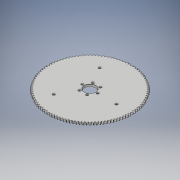
# Autodesk Inventor part: engrenage_rotation
Saved by Autodesk Inventor 2019 (Build 230136000, 136)
## iProperties
Created: 2018-05-17
Part Number: engrenage_rotation
Material: Générique
Document SubType Name: Modeling
Designer: Theo
Density: 1 g/cm^3
Appearance: Par défaut
Author: Theo
Autodesk Inventor part; units mm, degrees
ref_plane "YZ Plane" through (0, 0, 0) normal (1, 0, 0) x (0, 1, 0)
ref_plane "XZ Plane" through (0, 0, 0) normal (0, 1, 0) x (-1, 0, 0)
ref_plane "XY Plane" through (0, 0, 0) normal (0, 0, 1) x (1, 0, 0)
sketch "Esquisse1" plane through (0, 0, 0) normal (1, 0, 0) x (0, 1, 0)
  line L0 (-18.9677, 0) -> (18.9677, 0)
  line L1 (0, 99.5) -> (-0.5, 100)
  line L2 (-0.5, 100) -> (-4.5, 100)
  line L3 (-4.5, 100) -> (-5, 99.5)
  line L4 (-5, 99.5) -> (-5, 13.5)
  line L5 (0, 99.5) -> (0, 14)
  line L6 (-5, 13.5) -> (-0.5, 13.5)
  line L7 (0, 14) -> (-0.5, 13.5)
  point P0 (0, 0)
  point P1 (0, 0)
  dimension "d0" = 0.5
  dimension "d1" = 0.5
  dimension "d2" = 0.5
  dimension "d3" = 0.5
  dimension "d17" = 200
  dimension "d18" = 0.5
  dimension "d19" = 0.5
  dimension "d20" = 27
  dimension "d21" = 5
  constraints: 16 end point, 3 horizontal, 2 vertical, 1 coincident, 1 midpoint, 1 vertical alignment
  measures "d0" horizontal distance of L1.start L1.end
  measures "d1" horizontal distance of L1.start L1.end
  measures "d2" horizontal distance of L2.end L3.end
  measures "d3" horizontal distance of L2.end L3.end
  measures "d17" diameter of L2 L0
  measures "d18" horizontal distance of L5.end L6.end
  measures "d19" horizontal distance of L5.end L6.end
  measures "d20" diameter of L6 L0
  measures "d21" distance between parallel lines of L5 L4
revolve "Révolution1" add sketch "Esquisse1" angle 360 about axis through (0, -18.9677, 0) along (0, 1, 0)
sketch "Esquisse2" plane through (0, 0, 0) normal (0, 1, 0) x (1, 0, 0)
  point P0 (0, 0)
  point P1 (18.25, 0)
  point P2 (9.125, 15.805)
  point P3 (-9.125, 15.805)
  point P4 (-18.25, 0)
  point P5 (-9.125, -15.805)
  point P6 (9.125, -15.805)
  point P7 (63, 0)
  point P8 (-31.5, 54.5596)
  point P9 (-31.5, -54.5596)
  dimension "d23" = 18.25
  dimension "d26" = 360
  dimension "d44" = 63
  dimension "d47" = 360
  constraints: 2 horizontal alignment, 11 other
  measures "d23" distance of point (0, 0) point (18.25, 0)
  measures "d44" distance of point (63, 0) point (0, 0)
hole "Perçage1" at (18.25, 0, 0) at (9.125, 0, -15.805) at (-9.125, 0, -15.805) at (-18.25, 0, 0) at (-9.125, 0, 15.805) at (9.125, 0, 15.805) at (-31.5, 0, 54.5596) at (-31.5, 0, -54.5596) at (63, 0, 0) direction (0, -1, 0) diameter 4.2 end through all counterbore diameter 6 counterbore depth 2
sketch "Esquisse3" plane through (0, 0, 0) normal (0, 1, 0) x (1, 0, 0)
  line L0 (-2.43, -99.7088) -> (-0.433, -96.25)
  arc A0 (0.433, -96.25) -> (-0.433, -96.25) centre (0, -96.5) ccw
  line L1 (0.433, -96.25) -> (2.43, -99.7088)
  arc A1 (2.43, -99.7088) -> (2.8774, -99.9586) centre (2.863, -99.4588) ccw
  arc A2 (-2.8774, -99.9586) -> (-2.43, -99.7088) centre (-2.863, -99.4588) ccw
  circle A3 centre (0, 0) radius 100 projected
  circle A4 centre (0, 0) radius 99.5 projected
  circle A5 centre (-9.125, -15.805) radius 3 projected
  circle A6 centre (-9.125, 15.805) radius 3 projected
  circle A7 centre (18.25, 0) radius 3 projected
  circle A8 centre (9.125, 15.805) radius 3 projected
  circle A9 centre (-18.25, 0) radius 3 projected
  circle A10 centre (9.125, -15.805) radius 3 projected
  circle A11 centre (0, 0) radius 99.5 projected
  circle A12 centre (0, 0) radius 14 projected
  point P0 (0, 0)
  point P1 (0, -100)
  dimension "d35" = 0.5
  dimension "d36" = 0.5
  dimension "d38" = 60
  dimension "d49" = 3.5
  constraints: 9 point on circle, 6 tangent, 4 end point, 3 centre point, 2 vertical alignment, 1 equal length, 1 equal radius, 1 other
  measures "d35" radius of A0
  measures "d36" radius of A2
  measures "d38" angle of L1 L0
  measures "d49" distance of point (0, -100) A0.centre
extrude "Extrusion1" cut sketch "Esquisse3" against normal up to surface (5 mm away) contours L0 A4 L1 A1 A3 A2 | L0 A0 L1 A4 picked at (0.2549, -99.8293) picked at (1.164, -98.4069)
pattern_circular "Réseau circulaire1" count 108 over 360 about axis through (0, -10, 0) along (0, 1, 0) of "Extrusion1"
equation "\"d0\" = d6"
equation "\"d1\" = d6"
equation "\"d2\" = d6"
equation "\"d3\" = d6"
equation "\"d19\" = d18"
equation "\"d6\" = 0.5"
